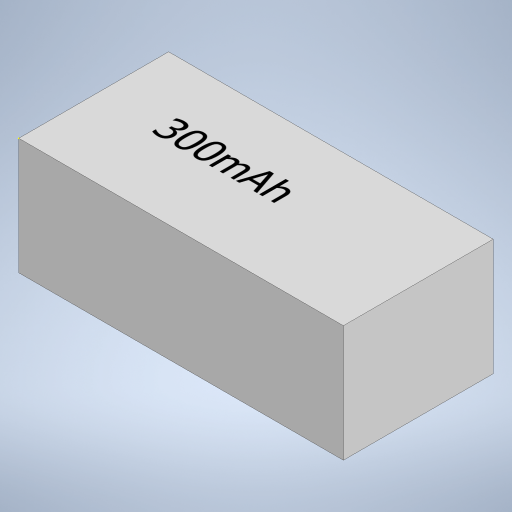
# Autodesk Inventor part: lipo-300
Saved by Autodesk Inventor 2023.5 (Build 275446000, 446)
## iProperties
Created: 2025-03-17
Part Number: lipo-300
Material: Ogólny
Document SubType Name: Modeling
Designer: kamil
Density: 1 g/cm^3
Appearance: Domyślna
Author: kamil
Autodesk Inventor part; units mm, degrees
ref_plane "YZ Plane" through (0, 0, 0) normal (1, 0, 0) x (0, 1, 0)
ref_plane "XZ Plane" through (0, 0, 0) normal (0, 1, 0) x (-1, 0, 0)
ref_plane "XY Plane" through (0, 0, 0) normal (0, 0, 1) x (1, 0, 0)
sketch "Szkic1" plane through (0, 0, 0) normal (0, 1, 0) x (-1, 0, 0)
  line L0 (0, 0) -> (-39, 0)
  line L1 (-39, 0) -> (-39, -18)
  line L2 (-39, -18) -> (0, -18)
  line L3 (0, -18) -> (0, 0)
  dimension "d0" = 39
  dimension "d1" = 18
  constraints: 8 end point, 2 parallel, 1 horizontal, 1 perpendicular
  measures "d0" distance of L2.end L1.end
  measures "d1" distance of L1.end L0.end
extrude "Wyciągnięcie proste1" add sketch "Szkic1" along normal blind 14
sketch "Szkic2" plane through (0, 14, 0) normal (0, 1, 0) x (1, 0, 0)
  line L0 (7.0982, 11.7973) -> (24.982, 11.7973) construction
  line L1 (24.982, 11.7973) -> (24.982, 5.0178) construction
  line L2 (24.982, 5.0178) -> (7.0982, 5.0178) construction
  line L3 (7.0982, 5.0178) -> (7.0982, 11.7973) construction
  point P0 (0, 0)
  constraints: 2 other
